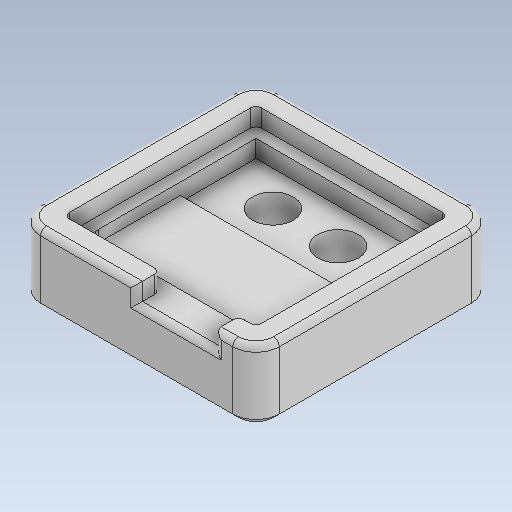
# Autodesk Inventor part: Light Pipe Mount - Top
Saved by Autodesk Inventor 2025 (Build 290162000, 162)
## iProperties
Created: 2024-06-14
Part Number: Light Pipe Mount - Top
Material: Generic
Document SubType Name: Modeling
Designer: ejohn
Density: 1 g/cm^3
Appearance: Default
Author: ejohn
Autodesk Inventor part; units mm, degrees
ref_plane "YZ Plane" through (0, 0, 0) normal (1, 0, 0) x (0, 1, 0)
ref_plane "XZ Plane" through (0, 0, 0) normal (0, 1, 0) x (-1, 0, 0)
ref_plane "XY Plane" through (0, 0, 0) normal (0, 0, 1) x (1, 0, 0)
sketch "Sketch1" plane through (0, 0, 0) normal (0, 1, 0) x (-1, 0, 0)
  line L0 (8, 8) -> (-8, 8) construction
  line L1 (-8, 8) -> (-8, -8) construction
  line L2 (-8, -8) -> (8, -8) construction
  line L3 (8, -8) -> (8, 8) construction
  line L4 (8, 8) -> (-8, -8) construction
  line L5 (-8, 8) -> (8, -8) construction
  line L6 (-8.25, 8.25) -> (8.25, 8.25)
  line L7 (8.25, 8.25) -> (8.25, -8.25)
  line L8 (8.25, -8.25) -> (-8.25, -8.25)
  line L9 (-8.25, -8.25) -> (-8.25, 8.25)
  line L10 (-8.25, 8.25) -> (8.25, -8.25) construction
  line L11 (8.25, 8.25) -> (-8.25, -8.25) construction
  line L12 (-10.25, 10.25) -> (10.25, 10.25)
  line L13 (10.25, 10.25) -> (10.25, -10.25)
  line L14 (10.25, -10.25) -> (-10.25, -10.25)
  line L15 (-10.25, -10.25) -> (-10.25, 10.25)
  line L16 (-10.25, 10.25) -> (10.25, -10.25) construction
  line L17 (10.25, 10.25) -> (-10.25, -10.25) construction
  circle A0 centre (2.8, -4.25) radius 1.75
  circle A1 centre (-2.8, -4.25) radius 1.75
  line L18 (7.25, -7.25) -> (-7.25, -7.25)
  line L19 (-7.25, -1.25) -> (7.25, -1.25)
  line L20 (7.25, -1.25) -> (7.25, -7.25)
  line L21 (-7.25, -1.25) -> (-7.25, -7.25)
  line L22 (-6.75, 8.25) -> (-6.75, 10.25)
  line L23 (0, 8.25) -> (0, 10.25)
  point P0 (0, 0)
  point P1 (0, -1.25)
  point P2 (7.25, -4.25)
  dimension "d0" = 16
  dimension "d1" = 16.5
  dimension "d2" = 2
  dimension "d3" = 3.5
  dimension "d4" = 5.6
  dimension "d5" = 2.8
  dimension "d6" = 6
  dimension "d7" = 1
  dimension "d8" = 1
  dimension "d15" = 1.5
  constraints: 48 end point, 10 midpoint, 7 parallel, 5 horizontal, 5 perpendicular, 4 point on line, 2 centre point, 2 horizontal alignment, 2 vertical, 1 equal radius, 1 vertical alignment
  measures "d0" distance of L1.end L2.end
  measures "d1" distance of L7.end L8.end
  measures "d2" distance between parallel lines of L8 L14
  measures "d3" diameter of A0
  measures "d4" distance of A1.centre A0.centre
  measures "d5" horizontal distance of point (0, 0) A0.centre
  measures "d6" distance of L19.end L18.start
  measures "d7" distance between parallel lines of L18 L8
  measures "d8" distance between parallel lines of L20 L7
  measures "d15" distance between parallel lines of L22 L9
extrude "Extrusion1" add sketch "Sketch1" along normal blind 1.5 contours L9 L8 L7 L6 L23 L12 L13 L14 L15 L22
extrude "Extrusion2" add sketch "Sketch1" against normal blind 1.5 contours L9 L8 L7 L6 L23 L12 L13 L14 L15 L22 | L6 L7 L8 L9 | L22 L12 L23 L6
sketch "Sketch2" plane through (0, -1.5, 0) normal (0, -1, 0) x (1, 0, 0)
  line L0 (-10.25, -10.25) -> (10.25, -10.25) projected
  line L1 (10.25, -10.25) -> (10.25, 10.25) projected
  line L2 (10.25, 10.25) -> (-10.25, 10.25) projected
  line L3 (-10.25, 10.25) -> (-10.25, -10.25) projected
  line L4 (-7.25, -1.25) -> (7.25, -1.25) projected
  line L5 (7.25, -1.25) -> (7.25, -7.25) projected
  line L6 (7.25, -7.25) -> (-7.25, -7.25) projected
  line L7 (-7.25, -7.25) -> (-7.25, -1.25) projected
  circle A0 centre (2.8, -4.25) radius 1.75 projected
  circle A1 centre (-2.8, -4.25) radius 1.75 projected
  point P0 (0, 0)
extrude "Extrusion3" add sketch "Sketch2" along normal blind 3 contours L3 L2 L1 L0 | L4 L5 L6 L7
fillet "Fillet2" radius 2 4 edges at (-10.25, -1.5, 10.25) (-10.25, -1.5, -10.25) (10.25, -1.5, -10.25) (10.25, -1.5, 10.25)
fillet "Fillet3" radius 0.5 18 edges at (-9.6642, 1.5, 9.6642) (-4.125, 1.5, 10.25) (-9.6642, 1.5, -9.6642) (0, 1.5, -10.25) (9.6642, 1.5, -9.6642) (10.25, 1.5, 0) (9.6642, 1.5, 9.6642) (7.5, 1.5, 10.25) (-10.25, 1.5, 0) (0, 0.75, 10.25) (3.375, 0, 10.25) (6.75, 0.75, 10.25) (-8.25, 0.75, 8.25) (-8.25, 0.75, -8.25) (8.25, 0.75, -8.25) (8.25, 0.75, 8.25) (6.75, 0.75, 8.25) (0, 0.75, 8.25)
chamfer "Chamfer1" distance 0.5 angle 45 10 edges at (1.05, -4.5, -4.25) (-4.55, -4.5, -4.25) (0, -4.5, 10.25) (-9.6642, -4.5, 9.6642) (-10.25, -4.5, 0) (-9.6642, -4.5, -9.6642) (0, -4.5, -10.25) (9.6642, -4.5, -9.6642) (10.25, -4.5, 0) (9.6642, -4.5, 9.6642)
sketch "Sketch3" plane through (0, 0, 0) normal (0, 1, 0) x (1, 0, 0)
  line L0 (7.25, 1.25) -> (-7.25, 1.25) projected
  line L1 (-7.25, 1.25) -> (-7.25, 7.25) projected
  line L2 (-7.25, 7.25) -> (7.25, 7.25) projected
  line L3 (7.25, 7.25) -> (7.25, 1.25) projected
  arc A0 (7.75, -8.25) -> (8.25, -7.75) centre (7.75, -7.75) ccw projected
  line L4 (8.25, 7.75) -> (8.25, -7.75) projected
  arc A1 (8.25, 7.75) -> (7.75, 8.25) centre (7.75, 7.75) ccw projected
  line L5 (-7.75, 8.25) -> (7.75, 8.25) projected
  arc A2 (-7.75, 8.25) -> (-8.25, 7.75) centre (-7.75, 7.75) ccw projected
  line L6 (-8.25, -7.75) -> (-8.25, 7.75) projected
  arc A3 (-8.25, -7.75) -> (-7.75, -8.25) centre (-7.75, -7.75) ccw projected
  line L7 (-0.5, -8.25) -> (-7.75, -8.25) projected
  arc A4 (0, -8.75) -> (-0.5, -8.25) centre (-0.5, -8.75) ccw projected
  line L8 (0, -9.75) -> (0, -8.75) projected
  line L9 (6.75, -9.75) -> (0, -9.75) projected
  line L10 (6.75, -8.75) -> (6.75, -9.75) projected
  arc A5 (7.25, -8.25) -> (6.75, -8.75) centre (7.25, -8.75) ccw projected
  line L11 (7.75, -8.25) -> (7.25, -8.25) projected
  line L12 (-7.25, 1.25) -> (7.25, 1.25)
  line L13 (7.25, 1.25) -> (7.25, -7.25)
  line L14 (7.25, -7.25) -> (-7.25, -7.25)
  line L15 (-7.25, -7.25) -> (-7.25, 1.25)
  point P0 (0, 0)
  dimension "d22" = 1
  constraints: 8 end point, 2 parallel, 1 horizontal, 1 perpendicular
  measures "d22" distance between parallel lines of L14 L7
extrude "Extrusion4" cut sketch "Sketch3" against normal blind 1 contours L13 L14 L15 L0
chamfer "Chamfer2" distance 0.5 angle 45 1 edges at (0, -1, -1.25)
fillet "Fillet4" radius 1 2 edges at (-7.25, -0.5, 7.25) (7.25, -0.5, 7.25)
equation "\"d5\" = 0.5 * d4"
equation "\"d8\" = d7"
body "Solid1"
